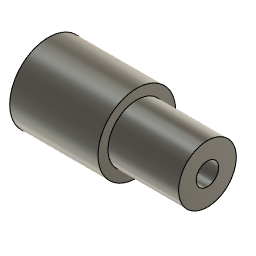
pieza motor para impresion 3D v1 (Autodesk Fusion 360 design; units mm, degrees)
Autodesk Fusion 360 part; units mm, degrees
sketch "Boceto1" plane through (0, 0, 0) normal (1, 0, 0) x (0, 1, 0)
  circle A0 centre (4.4228, -4.6349) radius 3.175
  circle A1 centre (4.4228, -4.6349) radius 8.175
  dimension "d1" = 6.35
  dimension "d2" = 5
  measures "d1" diameter of A0
extrude "Extruir1" add sketch "Boceto1" along normal blind 15
sketch "Boceto2" plane through (0, 0, 0) normal (-1, 0, 0) x (0, -1, 0)
  circle A0 centre (-4.4228, -4.6349) radius 3.175
  circle A1 centre (-4.4228, -4.6349) radius 8.175
  circle A2 centre (-4.4228, -4.6349) radius 8.175
  constraint concentric A0 A2
extrude "Extruir2" add sketch "Boceto2" along normal blind 5 contours A0 | A1 A2
sketch "Boceto3" plane through (-5, 0, 0) normal (-1, 0, 0) x (0, -1, 0)
  circle A0 centre (-4.4228, -4.6349) radius 8.175
  circle A1 centre (-4.4228, -4.6349) radius 11
  dimension "d7" = 22
  constraint concentric A0 A1
  measures "d7" diameter of A1
extrude "Extruir3" add sketch "Boceto3" along normal blind 25 contours A0 | A1
sketch "Boceto4" plane through (-30, 0, 0) normal (-1, 0, 0) x (0, -1, 0)
  circle A0 centre (-4.4228, -4.6349) radius 11
  circle A1 centre (-4.4228, -4.6349) radius 6
  dimension "d10" = 12
  constraint concentric A0 A1
  measures "d10" diameter of A1
extrude "Extruir4" cut sketch "Boceto4" against normal blind 23 contours A1
